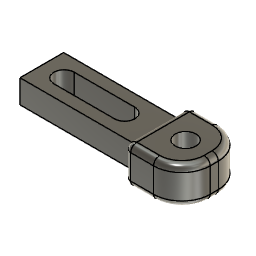
Bowflex C7 (Autodesk Fusion 360 design; units mm, degrees)
Autodesk Fusion 360 part; units mm, degrees
note: some values were not read from the file. Set by a fixed rule: which sketch regions a step uses.
sketch "Sketch4" plane through (0, 0, 9.1) normal (0, 0, 1) x (-1, 0, 0)
  circle A0 centre (-42, -8) radius 2.5
  line L0 (-50, 0) -> (-50, -16)
  line L1 (-50, -16) -> (-21.5, -16)
  line L2 (-21.5, -16) -> (-21.5, 0)
  line L3 (-21.5, 0) -> (-50, 0)
  line L4 (-45.9833, -10.338) -> (-41.9669, -12.6187)
  line L5 (-41.9669, -12.6187) -> (-37.9835, -10.2807)
  line L6 (-37.9835, -10.2807) -> (-38.0167, -5.662)
  line L7 (-38.0167, -5.662) -> (-42.0331, -3.3813)
  line L8 (-42.0331, -3.3813) -> (-46.0165, -5.7193)
  line L9 (-46.0165, -5.7193) -> (-45.9833, -10.338)
  point P0 (-42, -8)
  dimension "d65" = 4
  constraint coincident P0 A0.centre
  measures "d65" distance of P0 L9
sketch "Sketch1" plane through (0, 0, 0) normal (0, 0, 1) x (1, 0, 0)
  line L0 (21.5, 0) -> (50, 0)
  line L1 (50, 0) -> (50, 16)
  line L2 (50, 16) -> (21.5, 16)
  line L3 (21.5, 8) -> (50, 8)
  line L4 (21.5, 16) -> (21.5, 8)
  line L5 (21.5, 0) -> (21.5, 8)
  circle A0 centre (27, 8) radius 2.5
  circle A1 centre (42, 8) radius 2.5
  line L6 (21.5, 13.5) -> (50, 13.5)
  line L7 (21.5, 2.5) -> (50, 2.5)
  line L8 (27, 10.5) -> (27, 5.5) construction
  line L9 (42, 10.5) -> (42, 5.5) construction
  line L10 (27, 10.5) -> (42, 10.5)
  line L11 (27, 5.5) -> (42, 5.5)
  line L12 (50, 8) -> (62.5333, 8)
  circle A2 centre (57.075, 8) radius 2.575
  line L13 (57.075, 8) -> (57.075, 16) construction
  line L14 (57.075, 8) -> (57.075, 0) construction
  line L15 (50, 0) -> (57.075, 0)
  line L16 (54.5, 8) -> (54.5, 0)
  line L17 (50, 16) -> (57.075, 16)
  line L18 (64.15, 16) -> (57.075, 16)
  line L19 (59.65, 8) -> (59.65, 0)
  line L20 (64.15, 0) -> (57.075, 0)
  line L21 (64.15, 0) -> (64.15, 16)
  dimension "d1_1" = 50
  dimension "d8_1" = 5
  dimension "d10_1" = 5
  dimension "d11_1" = 8
  dimension "d12_1" = 2.5
  dimension "d35_1" = 15
  dimension "d36_1" = 5.5
  dimension "d53_1" = 5.15
  dimension "d54_1" = 7.075
  constraint horizontal L0
  constraint vertical L1
  constraint horizontal L2
  constraint midpoint L1 L3.end
  constraint perpendicular L3 L4
  constraint perpendicular L3 L5
  constraint coincident L3 A0.centre
  constraint coincident L3 A1.centre
  constraint coincident L4 L6.start
  constraint coincident L1 L6.end
  constraint perpendicular L1 L6
  constraint symmetric L3 L6.start L7.start
  constraint symmetric L3 L6.end L7.end
  constraint coincident A0 L8.start
  constraint coincident A0 L8.end
  constraint perpendicular L3 L8
  constraint coincident A1 L9.start
  constraint coincident A1 L9.end
  constraint perpendicular L3 L9
  constraint tangent A1 L10
  constraint symmetric L3 L8.start L8.end
  constraint symmetric L3 L9.start L9.end
  constraint perpendicular L1 L12
  constraint coincident L12 A2.centre
  constraint coincident A2.centre L13.start
  constraint perpendicular L2 L13
  constraint perpendicular L0 L14
  constraint perpendicular L14 L15
  constraint coincident A2 L16.start
  constraint coincident L12 L16.start
  constraint coincident L15 L16.end
  constraint tangent A2 L16
  constraint perpendicular L13 L17
  constraint symmetric L0.end L13 L20.start
  constraint symmetric L1.end L13 L18.start
  constraint symmetric L17.end L13 L18.end
  constraint symmetric L13 L14.end L15.end
  constraint symmetric L13 L16.start L19.start
  constraint symmetric L13 L16.end L19.end
  measures "d1_1" distance of origin L0.end
  measures "d8_1" diameter of A0
  measures "d10_1" diameter of A1
  measures "d11_1" distance of L1 A1.centre
  measures "d12_1" distance of L2 L6
  measures "d35_1" distance of A0.centre A1.centre
  measures "d36_1" distance of L5 A0.centre
  measures "d53_1" diameter of A2
  measures "d54_1" distance of L3.end A2.centre
extrude "Extrude1" add sketch "Sketch1" along normal blind 9.1 contours L0 L1 L5 L7 | L1 L3 L5 A0 A1 L7 L11 | L1 L3 L4 A0 A1 L6 L10 | L3 A0 | L3 A0 | L1 L2 L4 L6 | L3 A0 A1 L10 | L3 A0 A1 L11 makes body 1
extrude "Extrude2" cut sketch "Sketch1" along normal blind 5.9 contours L1 L3 L5 A0 A1 L7 L11 | L1 L3 L4 A0 A1 L6 L10 | L3 A0 | L3 A0 | L3 A0 A1 L10 | L3 A0 A1 L11 bodies 1
extrude "Extrude3" add sketch "Sketch1" along normal blind 5.8 separate body contours L1 L3 L5 A0 A1 L7 L11 | L1 L3 L4 A0 A1 L6 L10 makes body 2
extrude "Extrude9" add sketch "Sketch1" against normal blind 3.1 contours L0 L1 L5 L7 | L1 L3 L5 A0 A1 L7 L11 | L1 L3 L4 A0 A1 L6 L10 | L3 A0 | L3 A0 | L1 L2 L4 L6 | L3 A1 | L3 A1 | L3 A0 A1 L10 | L3 A0 A1 L11 bodies 1
extrude "Extrude10" cut sketch "Sketch1" against normal blind 0.1 contours L1 L3 L5 A0 A1 L7 L11 | L1 L3 L4 A0 A1 L6 L10 | L3 A0 | L3 A0 | L3 A1 | L3 A1 | L3 A0 A1 L10 | L3 A0 A1 L11 bodies 1
move_face "OffsetFaces1" offset -0.1 2 faces at (40.5, 13.5, 1.9333) (40.5, 2.5, 1.9333) on bodies 2
extrude "Extrude6" add sketch "Sketch1" along normal blind 7.55 contours L1 L12 L15 L16 | A2 L15 L16 L19 L20 | L1 L12 A2 L17 L18 L19 L20 L21 bodies 2
extrude "Extrude12" add sketch "Sketch1" against normal blind 1.55 contours L1 L12 L15 L16 | A2 L15 L16 L19 L20 | L1 L12 A2 L17 L18 L19 L20 L21 bodies 2
extrude "Extrude14" cut sketch "Sketch1" against normal blind 3.1 contours L3 A1 | L3 A1 bodies 1
move_body "Move1" bodies 2 to x (1, 0, 0) y (0, 1, 0) z (0, 0, 1) at (13, 0, 0)
extrude "Extrude11" cut sketch "Sketch4" against normal blind 0.75 contours L4 L5 L6 L7 L8 L9 bodies 1
fillet "Fillet3" radius 1.5 6 edges at (35.75, 16, 9.1) (35.75, 16, -3.1) (35.75, 0, 9.1) (35.75, 0, -3.1) (50, 0, 3) (50, 16, 3) on bodies 1 2
fillet "Fillet3" radius 4 2 edges at (50, 8, 9.1) (50, 8, -3.1) on bodies 1 2
fillet "Fillet3" radius 1.5 10 edges at (70.075, 0, 7.55) (70.075, 0, -1.55) (63, 8, -1.55) (63, 0, 3) (63, 8, 7.55) (63, 16, 3) (70.075, 16, -1.55) (70.075, 16, 7.55) (77.15, 8, 7.55) (77.15, 8, -1.55) on bodies 1 2
fillet "Fillet3" radius 7 2 edges at (77.15, 0, 3) (77.15, 16, 3) on bodies 1 2
delete_body "RemoveBody1" bodies 1
move_body "Move2" bodies 2 to x (1, 0, 0) y (0, 1, 0) z (0, 0, 1) at (-12, 0, 0)
equation "d29 = ( 3.1 / 2 ) * 1 mm + 6 mm"
equation "d54_1 = 4.5 mm + ( 5.15 / 2 ) * 1 mm"
equation "d252 = -9.1 mm + 6 mm"
equation "d259 = ( -3.1 / 2 ) * 1 mm"
